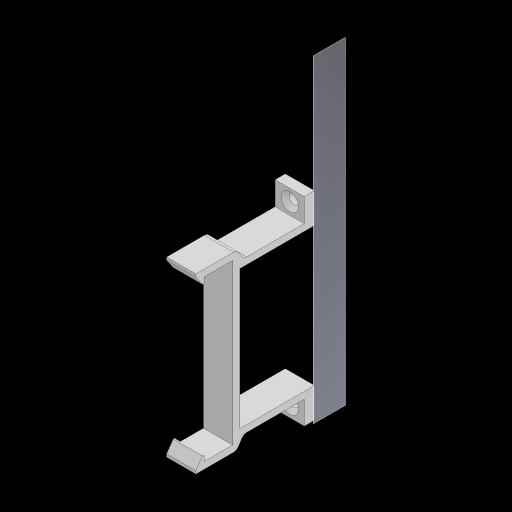
# Autodesk Inventor part: batteryHolder
Saved by Autodesk Inventor 2024.3 (Build 283343010, 343A)
## iProperties
Created: 2025-04-14
Part Number: batteryHolder
Material: Generic
Document SubType Name: Modeling
Designer: Oleg Kelner
Density: 1 g/cm^3
Appearance: Default
Author: Oleg Kelner
Autodesk Inventor part; units mm, degrees
ref_plane "YZ Plane" through (0, 0, 0) normal (1, 0, 0) x (0, 1, 0)
ref_plane "XZ Plane" through (0, 0, 0) normal (0, 1, 0) x (-1, 0, 0)
ref_plane "Work Plane4" through (-45.25, 257.5287, -0.5) normal (1, 0, 0) x (0, -1, 0)
sketch "Sketch5" plane through (-45.25, 257.5287, -0.5) normal (1, 0, 0) x (0, -1, 0)
  line L0 (45.7104, -25.5535) -> (92.7104, -25.5535)
  line L1 (92.7104, -25.5535) -> (92.7104, -0.0535)
  line L2 (45.7104, -0.0535) -> (45.7104, -25.5535)
  line L3 (95.2104, -28.0535) -> (43.2104, -28.0535)
  line L4 (43.2104, -28.0535) -> (43.2104, -3.5535)
  line L5 (103.2104, -0.0535) -> (103.2104, -3.5535)
  line L6 (103.2104, -3.5535) -> (95.2104, -3.5535)
  line L7 (92.7104, -0.0535) -> (103.2104, -0.0535)
  line L8 (95.2104, -3.5535) -> (95.2104, -28.0535)
  line L9 (43.2104, -3.5535) -> (35.2104, -3.5535)
  line L10 (35.2104, -3.5535) -> (35.2104, -0.0535)
  line L11 (45.7104, -0.0535) -> (35.2104, -0.0535)
  point P0 (257.5287, -0.5)
  dimension "d10" = 2.5
  dimension "d11" = 3.5
  dimension "d12" = 2.5
  dimension "d13" = 8
  dimension "d14" = 2.5
  dimension "d17" = 8
  dimension "d40" = 47
  dimension "d41" = 25.5
  constraints: 24 end point, 3 vertical, 2 collinear, 1 horizontal, 1 perpendicular, 1 other
  measures "d10" distance between parallel lines of L0 L3
  measures "d11" distance between parallel lines of L7 L6
  measures "d12" distance between parallel lines of L1 L8
  measures "d13" distance between parallel lines of L8 L5
  measures "d14" distance between parallel lines of L4 L2
  measures "d17" distance between parallel lines of L10 L4
  measures "d40" distance between parallel lines of L2 L1
  measures "d41" distance between parallel lines of L7 L0
extrude "Extrusion2" add sketch "Sketch5" against normal blind 10
sketch "Sketch6" plane through (-45.25, 154.3183, 3.0535) normal (0, 0, 1) x (1, 0, 0)
  line L0 (0, 68) -> (0, 60) projected
  line L1 (0, 68) -> (-10, 68) projected
  line L2 (-10, 60) -> (-10, 68) projected
  line L3 (0, 60) -> (-10, 60) projected
  line L4 (0, 8) -> (0, 0) projected
  line L5 (0, 8) -> (-10, 8) projected
  line L6 (-10, 0) -> (-10, 8) projected
  line L7 (0, 0) -> (-10, 0) projected
  line L8 (-10, 68) -> (0, 60) construction
  line L9 (0, 68) -> (-10, 60) construction
  line L10 (0, 8) -> (-10, 8) construction
  line L11 (-10, 8) -> (0, 0) construction
  line L12 (0, 8) -> (-10, 0) construction
  point P0 (45.25, -154.3183)
  point P1 (-5, 64)
  point P2 (-5, 4)
  constraints: 8 end point, 2 midpoint, 2 parallel
hole "Hole1" at (-50.25, 218.3183, 3.0535) at (-50.25, 158.3183, 3.0535) direction (0, 0, -1) diameter 3.2 end through all countersink diameter 6 countersink angle 90
sketch "Sketch7" plane through (-55.25, 257.5287, -0.5) normal (-1, 0, 0) x (0, 0, 1)
  line L0 (37.6535, -68.1104) -> (35.0535, -68.1104) projected
  line L1 (35.0535, -68.1104) -> (35.0535, -70.3104) projected
  line L2 (35.0535, -70.3104) -> (37.6535, -70.3104) projected
  line L3 (37.6535, -70.3104) -> (37.6535, -96.3604) projected
  line L4 (37.6535, -96.3604) -> (28.0535, -96.3604) projected
  line L5 (28.0535, -96.3604) -> (28.0535, -42.0604) projected
  line L6 (37.6535, -42.0604) -> (28.0535, -42.0604) construction
  line L7 (37.6535, -42.0604) -> (37.6535, -68.1104) construction
  line L8 (37.6535, -44.5604) -> (40.6535, -44.5604)
  line L9 (40.6535, -44.5604) -> (40.6535, -39.5604)
  line L10 (40.6535, -39.5604) -> (26.6535, -39.5604)
  line L11 (26.6535, -39.5604) -> (24.4035, -43.2104)
  line L12 (3.5535, -43.2104) -> (28.0535, -43.2104) projected
  line L13 (28.0535, -43.2104) -> (24.4035, -43.2104)
  line L14 (37.8535, -44.5604) -> (37.8535, -41.8604)
  line L15 (37.8535, -41.8604) -> (28.0535, -41.8604)
  line L16 (28.0535, -41.8604) -> (28.0535, -42.0604)
  point P0 (0.5, -257.5287)
  dimension "d42" = 2.5
  dimension "d43" = 3
  dimension "d44" = 5
  dimension "d45" = 3.65
  dimension "d46" = 14
  dimension "d47" = 9.6
  dimension "d48" = 3.65
  dimension "d49" = 0.2
  dimension "d50" = 0.2
  constraints: 16 end point, 3 perpendicular, 3 point on line, 2 horizontal, 1 collinear, 1 vertical
  measures "d42" distance between parallel lines of L6 L10
  measures "d43" distance between parallel lines of L9 L7
  measures "d44" distance between parallel lines of L8 L10
  measures "d45" distance from line of L5 L11.end
  measures "d46" distance of L9.end L10.end
  measures "d47" distance between parallel lines of L7 L5
  measures "d48" distance between parallel lines of L12 L10
  measures "d49" distance between parallel lines of L14 L7
  measures "d50" distance between parallel lines of L15 L6
extrude "Extrusion3" add sketch "Sketch7" against normal blind 10
chamfer "Chamfer1" distance 4 distance2 2.8 1 edges at (-50.25, 212.9683, 40.1535) measured on face at (-51.9167, 214.6349, 40.1535)
fillet "Fillet2" radius 0.3 2 edges at (-50.25, 212.9683, 37.3536) (-50.25, 212.9683, 37.3535)
ref_plane "Work Plane5" through (-45.25, 188.3183, 3.0535) normal (0, -1, 0) x (1, 0, 0)
mirror "Mirror2" about plane through (-45.25, 188.3183, 3.0535) normal (0, -1, 0) of "Extrusion3", "Fillet2", "Chamfer1"
sketch "Sketch8" plane through (-45.25, 257.5287, -0.5) normal (1, 0, 0) x (0, 0, -1)
  line L0 (-25.5535, -45.7104) -> (-0.0535, -45.7104) projected
  line L1 (-25.5535, -45.7104) -> (-0.0535, -45.7104)
  line L2 (-0.0535, -45.7104) -> (-0.0535, -45.5104)
  line L3 (-0.0535, -45.5104) -> (-25.5535, -45.5104)
  line L4 (-25.5535, -45.5104) -> (-25.5535, -45.7104)
  line L5 (-0.0535, -92.7104) -> (-25.5535, -92.7104) projected
  line L6 (-25.5535, -92.7104) -> (-0.0535, -92.7104)
  line L7 (-0.0535, -92.7104) -> (-0.0535, -92.9104)
  line L8 (-0.0535, -92.9104) -> (-25.5535, -92.9104)
  line L9 (-25.5535, -92.9104) -> (-25.5535, -92.7104)
  point P0 (-0.5, -257.5287)
  dimension "d51" = 0.2
  dimension "d52" = 0.2
  constraints: 16 end point, 5 equal length, 3 perpendicular
  measures "d51" distance of L2.end L0.end
  measures "d52" distance of L5.start L7.end
extrude "Extrusion4" cut sketch "Sketch8" against normal through all
fillet "Fillet3" radius 2 4 edges at (-50.25, 217.9683, 26.1535) (-50.25, 214.3183, 23.9035) (-50.25, 158.6683, 26.1535) (-50.25, 162.3183, 23.9035)
equation "\"d12\" = d10"
equation "\"d14\" = d10"
equation "\"d17\" = d13"
equation "\"d45\" = d48"
body "Solid1"
body "Solid2"
